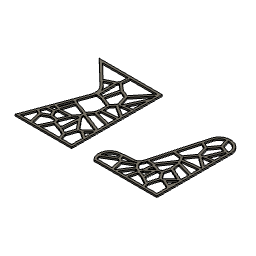
StrangeOutfit-Sides (Autodesk Fusion 360 design; units mm, degrees)
Autodesk Fusion 360 part; units mm, degrees
(part 1 of 2)
sketch "Sketch1" plane through (0, 0, 0) normal (0, 1, 0) x (1, 0, 0)
  line L0 (-508, 0) -> (0, 0)
  line L1 (-561.4783, 808.976) -> (-349.2633, 603.2383)
  arc A0 (-565.2203, 812.8) -> (-561.4783, 808.976) centre (-490.7581, 881.9227) ccw
  line L2 (-324.7055, 495.0118) -> (-508, 0)
  line L3 (0, 812.8) -> (-565.2203, 812.8)
  arc A1 (-349.2633, 603.2383) -> (-324.7055, 495.0118) centre (-419.9835, 530.2916) cw
  line L4 (0, 0) -> (0, 812.8)
  spline S0 degree 3 poles (197.1979, -94.8264) (181.7287, -81.3513) (181.7287, -81.3513) (184.3434, -52.8038) knots 0 0 0 0 1 1 1 1
  spline S1 degree 3 poles (184.3434, -52.8038) (186.9581, -24.2563) (186.9581, -24.2563) (221.5677, -24.2563) knots 0 0 0 0 1 1 1 1
  spline S2 degree 3 poles (221.5677, -24.2563) (256.1772, -24.2563) (256.1772, -24.2563) (249.4808, -61.402) knots 0 0 0 0 1 1 1 1
  spline S3 degree 3 poles (249.4808, -61.402) (242.7844, -98.5476) (242.7844, -98.5476) (227.7258, -103.4246) knots 0 0 0 0 1 1 1 1
  spline S4 degree 3 poles (227.7258, -103.4246) (212.6672, -108.3015) (212.6672, -108.3015) (197.1979, -94.8264) knots 0 0 0 0 1 1 1 1
  spline S5 degree 3 poles (314.1363, -605.8547) (333.9886, -586.6079) (333.9886, -586.6079) (347.2933, -588.796) knots 0 0 0 0 1 1 1 1
  spline S6 degree 3 poles (347.2933, -588.796) (360.598, -590.9842) (360.598, -590.9842) (371.6807, -608.3365) knots 0 0 0 0 1 1 1 1
  spline S7 degree 3 poles (371.6807, -608.3365) (382.7633, -625.6888) (382.7633, -625.6888) (369.5852, -652.1299) knots 0 0 0 0 1 1 1 1
  spline S8 degree 3 poles (369.5852, -652.1299) (356.4071, -678.5711) (356.4071, -678.5711) (332.329, -676.3297) knots 0 0 0 0 1 1 1 1
  spline S9 degree 3 poles (332.329, -676.3297) (308.2508, -674.0883) (308.2508, -674.0883) (301.2674, -649.5949) knots 0 0 0 0 1 1 1 1
  spline S10 degree 3 poles (301.2674, -649.5949) (294.284, -625.1014) (294.284, -625.1014) (314.1363, -605.8546) knots 0 0 0 0 1 1 1 1
  line L5 (314.1363, -605.8546) -> (314.1363, -605.8547)
  spline S11 degree 3 poles (325.2577, -150.3081) (324.2502, -141.4606) (324.2502, -141.4606) (337.2456, -127.0451) knots 0 0 0 0 1 1 1 1
  spline S12 degree 3 poles (337.2456, -127.0451) (350.2411, -112.6297) (350.2411, -112.6297) (372.3999, -109.9629) knots 0 0 0 0 1 1 1 1
  spline S13 degree 3 poles (372.3999, -109.9629) (394.5588, -107.2962) (394.5588, -107.2962) (414.281, -123.2421) knots 0 0 0 0 1 1 1 1
  spline S14 degree 3 poles (414.281, -123.2421) (434.0032, -139.1881) (434.0032, -139.1881) (430.6769, -158.3617) knots 0 0 0 0 1 1 1 1
  spline S15 degree 3 poles (430.6769, -158.3617) (427.3505, -177.5353) (427.3505, -177.5353) (401.8439, -188.2391) knots 0 0 0 0 1 1 1 1
  spline S16 degree 3 poles (401.8439, -188.2391) (376.3374, -198.943) (376.3374, -198.943) (351.3013, -179.0493) knots 0 0 0 0 1 1 1 1
  spline S17 degree 3 poles (351.3013, -179.0493) (326.2652, -159.1556) (326.2652, -159.1556) (325.2577, -150.3081) knots 0 0 0 0 1 1 1 1
  spline S18 degree 3 poles (356.0613, -480.7521) (387.4233, -481.317) (387.4233, -481.317) (397.359, -499.3064) knots 0 0 0 0 1 1 1 1
  spline S19 degree 3 poles (397.359, -499.3064) (407.2948, -517.2958) (407.2948, -517.2958) (386.1882, -543.2085) knots 0 0 0 0 1 1 1 1
  spline S20 degree 3 poles (386.1882, -543.2085) (365.0816, -569.1212) (365.0816, -569.1212) (351.2654, -566.8489) knots 0 0 0 0 1 1 1 1
  spline S21 degree 3 poles (351.2654, -566.8489) (337.4492, -564.5766) (337.4492, -564.5766) (323.3468, -539.9771) knots 0 0 0 0 1 1 1 1
  spline S22 degree 3 poles (323.3468, -539.9771) (309.2444, -515.3777) (309.2444, -515.3777) (316.9719, -497.7824) knots 0 0 0 0 1 1 1 1
  spline S23 degree 3 poles (316.9719, -497.7824) (324.6994, -480.1871) (324.6994, -480.1871) (356.0613, -480.752) knots 0 0 0 0 1 1 1 1
  line L6 (356.0613, -480.752) -> (356.0613, -480.7521)
  spline S24 degree 3 poles (387.6685, -660.8912) (400.7266, -634.6908) (400.7266, -634.6908) (423.4349, -636.471) knots 0 0 0 0 1 1 1 1
  spline S25 degree 3 poles (423.4349, -636.471) (446.1432, -638.2512) (446.1432, -638.2512) (456.0097, -663.7671) knots 0 0 0 0 1 1 1 1
  spline S26 degree 3 poles (456.0097, -663.7671) (465.8762, -689.283) (465.8762, -689.283) (457.4993, -699.4999) knots 0 0 0 0 1 1 1 1
  spline S27 degree 3 poles (457.4993, -699.4999) (449.1223, -709.7169) (449.1223, -709.7169) (419.0273, -708.316) knots 0 0 0 0 1 1 1 1
  spline S28 degree 3 poles (419.0273, -708.316) (388.9322, -706.9152) (388.9322, -706.9152) (381.7713, -697.0034) knots 0 0 0 0 1 1 1 1
  spline S29 degree 3 poles (381.7713, -697.0034) (374.6104, -687.0917) (374.6104, -687.0917) (387.6685, -660.8913) knots 0 0 0 0 1 1 1 1
  line L7 (387.6685, -660.8913) -> (387.6685, -660.8912)
  spline S30 degree 3 poles (404.7879, -382.8824) (386.9787, -364.4613) (386.9787, -364.4613) (396.7831, -338.1032) knots 0 0 0 0 1 1 1 1
  spline S31 degree 3 poles (396.7831, -338.1032) (406.5874, -311.7451) (406.5874, -311.7451) (427.3969, -309.3698) knots 0 0 0 0 1 1 1 1
  spline S32 degree 3 poles (427.3969, -309.3698) (448.2065, -306.9944) (448.2065, -306.9944) (464.4713, -324.5012) knots 0 0 0 0 1 1 1 1
  spline S33 degree 3 poles (464.4713, -324.5012) (480.7362, -342.0079) (480.7362, -342.0079) (466.7089, -368.8424) knots 0 0 0 0 1 1 1 1
  spline S34 degree 3 poles (466.7089, -368.8424) (452.6817, -395.6768) (452.6817, -395.6768) (437.6393, -398.4902) knots 0 0 0 0 1 1 1 1
  spline S35 degree 3 poles (437.6393, -398.4902) (422.597, -401.3035) (422.597, -401.3035) (404.7878, -382.8824) knots 0 0 0 0 1 1 1 1
  line L8 (404.7878, -382.8824) -> (404.7879, -382.8824)
  spline S36 degree 3 poles (185.1347, -753.5733) (182.1571, -789.0148) (182.1571, -789.0148) (149.5573, -789.0148) knots 0 0 0 0 1 1 1 1
  spline S37 degree 3 poles (149.5573, -789.0148) (116.9575, -789.0148) (116.9575, -789.0148) (114.8929, -752.1146) knots 0 0 0 0 1 1 1 1
  spline S38 degree 3 poles (114.8929, -752.1146) (112.8282, -715.2145) (112.8282, -715.2145) (113.8529, -714.1235) knots 0 0 0 0 1 1 1 1
  spline S39 degree 3 poles (113.8529, -714.1235) (114.8777, -713.0325) (114.8777, -713.0325) (147.0962, -711.0195) knots 0 0 0 0 1 1 1 1
  spline S40 degree 3 poles (147.0962, -711.0195) (179.3148, -709.0066) (179.3148, -709.0066) (183.7135, -713.5691) knots 0 0 0 0 1 1 1 1
  spline S41 degree 3 poles (183.7135, -713.5691) (188.1122, -718.1316) (188.1122, -718.1316) (185.1347, -753.5732) knots 0 0 0 0 1 1 1 1
  line L9 (185.1347, -753.5732) -> (185.1347, -753.5733)
  spline S42 degree 3 poles (398.2716, -56.4462) (390.271, -88.5918) (390.271, -88.5918) (370.6111, -90.9578) knots 0 0 0 0 1 1 1 1
  spline S43 degree 3 poles (370.6111, -90.9578) (350.9513, -93.3237) (350.9513, -93.3237) (340.7662, -58.8122) knots 0 0 0 0 1 1 1 1
  spline S44 degree 3 poles (340.7662, -58.8122) (330.581, -24.3006) (330.581, -24.3006) (368.4266, -24.3006) knots 0 0 0 0 1 1 1 1
  spline S45 degree 3 poles (368.4266, -24.3006) (406.2722, -24.3006) (406.2722, -24.3006) (398.2716, -56.4462) knots 0 0 0 0 1 1 1 1
  line L10 (398.2716, -56.4462) -> (398.2716, -56.4462)
  spline S46 degree 3 poles (321.4781, -406.2143) (332.5431, -384.0384) (332.5431, -384.0384) (352.3085, -380.8845) knots 0 0 0 0 1 1 1 1
  spline S47 degree 3 poles (352.3085, -380.8845) (372.0739, -377.7306) (372.0739, -377.7306) (389.7648, -396.0293) knots 0 0 0 0 1 1 1 1
  spline S48 degree 3 poles (389.7648, -396.0293) (407.4556, -414.3281) (407.4556, -414.3281) (397.2221, -437.6806) knots 0 0 0 0 1 1 1 1
  spline S49 degree 3 poles (397.2221, -437.6806) (386.9886, -461.0332) (386.9886, -461.0332) (356.2186, -460.479) knots 0 0 0 0 1 1 1 1
  spline S50 degree 3 poles (356.2186, -460.479) (325.4486, -459.9247) (325.4486, -459.9247) (317.9308, -444.1575) knots 0 0 0 0 1 1 1 1
  spline S51 degree 3 poles (317.9308, -444.1575) (310.4131, -428.3902) (310.4131, -428.3902) (321.4781, -406.2144) knots 0 0 0 0 1 1 1 1
  line L11 (321.4781, -406.2144) -> (321.4781, -406.2143)
  spline S52 degree 3 poles (264.9537, -529.8005) (293.6396, -524.3322) (293.6396, -524.3322) (307.4969, -548.5041) knots 0 0 0 0 1 1 1 1
  spline S53 degree 3 poles (307.4969, -548.5041) (321.3541, -572.676) (321.3541, -572.676) (301.097, -592.3153) knots 0 0 0 0 1 1 1 1
  spline S54 degree 3 poles (301.097, -592.3153) (280.8398, -611.9546) (280.8398, -611.9546) (257.4922, -604.1541) knots 0 0 0 0 1 1 1 1
  spline S55 degree 3 poles (257.4922, -604.1541) (234.1447, -596.3536) (234.1447, -596.3536) (235.2062, -565.8113) knots 0 0 0 0 1 1 1 1
  spline S56 degree 3 poles (235.2062, -565.8113) (236.2677, -535.2689) (236.2677, -535.2689) (264.9537, -529.8005) knots 0 0 0 0 1 1 1 1
  spline S57 degree 3 poles (380.3364, -237.5005) (384.7414, -214.6927) (384.7414, -214.6927) (409.0824, -204.478) knots 0 0 0 0 1 1 1 1
  spline S58 degree 3 poles (409.0824, -204.478) (433.4234, -194.2633) (433.4234, -194.2633) (450.4003, -212.6655) knots 0 0 0 0 1 1 1 1
  spline S59 degree 3 poles (450.4003, -212.6655) (467.377, -231.0678) (467.377, -231.0678) (456.5522, -258.126) knots 0 0 0 0 1 1 1 1
  spline S60 degree 3 poles (456.5522, -258.126) (445.7273, -285.1843) (445.7273, -285.1843) (424.898, -287.5619) knots 0 0 0 0 1 1 1 1
  spline S61 degree 3 poles (424.898, -287.5619) (404.0687, -289.9394) (404.0687, -289.9394) (390, -275.1238) knots 0 0 0 0 1 1 1 1
  spline S62 degree 3 poles (390, -275.1238) (375.9314, -260.3082) (375.9314, -260.3082) (380.3364, -237.5005) knots 0 0 0 0 1 1 1 1
  spline S63 degree 3 poles (518.1162, -109.8607) (490.6468, -105.3557) (490.6468, -105.3557) (487.0263, -64.3304) knots 0 0 0 0 1 1 1 1
  spline S64 degree 3 poles (487.0263, -64.3304) (483.4058, -23.305) (483.4058, -23.305) (514.4957, -23.305) knots 0 0 0 0 1 1 1 1
  spline S65 degree 3 poles (514.4957, -23.305) (545.5855, -23.305) (545.5855, -23.305) (545.5855, -68.8354) knots 0 0 0 0 1 1 1 1
  spline S66 degree 3 poles (545.5855, -68.8354) (545.5855, -114.3657) (545.5855, -114.3657) (518.1162, -109.8607) knots 0 0 0 0 1 1 1 1
  spline S67 degree 3 poles (441.522, -418.9688) (457.0203, -416.0701) (457.0203, -416.0701) (483.5167, -439.8327) knots 0 0 0 0 1 1 1 1
  spline S68 degree 3 poles (483.5167, -439.8327) (510.0132, -463.5952) (510.0132, -463.5952) (483.0172, -488.7104) knots 0 0 0 0 1 1 1 1
  spline S69 degree 3 poles (483.0172, -488.7104) (456.0211, -513.8256) (456.0211, -513.8256) (440.5191, -510.3742) knots 0 0 0 0 1 1 1 1
  spline S70 degree 3 poles (440.5191, -510.3742) (425.0171, -506.9227) (425.0171, -506.9227) (414.9062, -488.6162) knots 0 0 0 0 1 1 1 1
  spline S71 degree 3 poles (414.9062, -488.6162) (404.7954, -470.3098) (404.7954, -470.3098) (415.4095, -446.0886) knots 0 0 0 0 1 1 1 1
  spline S72 degree 3 poles (415.4095, -446.0886) (426.0237, -421.8674) (426.0237, -421.8674) (441.522, -418.9688) knots 0 0 0 0 1 1 1 1
  spline S73 degree 3 poles (474.2518, -266.1599) (484.6175, -240.2495) (484.6175, -240.2495) (513.0731, -237.6245) knots 0 0 0 0 1 1 1 1
  spline S74 degree 3 poles (513.0731, -237.6245) (541.5287, -234.9996) (541.5287, -234.9996) (541.5287, -279.1463) knots 0 0 0 0 1 1 1 1
  spline S75 degree 3 poles (541.5287, -279.1463) (541.5287, -323.293) (541.5287, -323.293) (518.2971, -324.4617) knots 0 0 0 0 1 1 1 1
  spline S76 degree 3 poles (518.2971, -324.4617) (495.0655, -325.6304) (495.0655, -325.6304) (479.4758, -308.8504) knots 0 0 0 0 1 1 1 1
  spline S77 degree 3 poles (479.4758, -308.8504) (463.8861, -292.0704) (463.8861, -292.0704) (474.2518, -266.1599) knots 0 0 0 0 1 1 1 1
  spline S78 degree 3 poles (532.861, -454.3391) (519.4812, -454.2704) (519.4812, -454.2704) (492.0593, -429.6779) knots 0 0 0 0 1 1 1 1
  spline S79 degree 3 poles (492.0593, -429.6779) (464.6374, -405.0854) (464.6374, -405.0854) (479.5946, -376.472) knots 0 0 0 0 1 1 1 1
  spline S80 degree 3 poles (479.5946, -376.472) (494.5517, -347.8586) (494.5517, -347.8586) (520.3962, -346.5584) knots 0 0 0 0 1 1 1 1
  spline S81 degree 3 poles (520.3962, -346.5584) (546.2408, -345.2582) (546.2408, -345.2582) (546.2408, -399.833) knots 0 0 0 0 1 1 1 1
  spline S82 degree 3 poles (546.2408, -399.833) (546.2408, -454.4078) (546.2408, -454.4078) (532.861, -454.3391) knots 0 0 0 0 1 1 1 1
  line L12 (532.861, -454.3391) -> (532.861, -454.3391)
  spline S83 degree 3 poles (287.1401, -246.3243) (272.1959, -224.4344) (272.1959, -224.4344) (294.6473, -198.5119) knots 0 0 0 0 1 1 1 1
  spline S84 degree 3 poles (294.6473, -198.5119) (317.0987, -172.5894) (317.0987, -172.5894) (340.9663, -191.5547) knots 0 0 0 0 1 1 1 1
  spline S85 degree 3 poles (340.9663, -191.5547) (364.834, -210.5199) (364.834, -210.5199) (360.4335, -233.3043) knots 0 0 0 0 1 1 1 1
  spline S86 degree 3 poles (360.4335, -233.3043) (356.033, -256.0887) (356.033, -256.0887) (329.0586, -262.1515) knots 0 0 0 0 1 1 1 1
  spline S87 degree 3 poles (329.0586, -262.1515) (302.0843, -268.2142) (302.0843, -268.2142) (287.1401, -246.3243) knots 0 0 0 0 1 1 1 1
  spline S88 degree 3 poles (165.1478, -50.93) (162.5663, -79.1146) (162.5663, -79.1146) (135.0164, -86.2518) knots 0 0 0 0 1 1 1 1
  spline S89 degree 3 poles (135.0164, -86.2518) (107.4664, -93.389) (107.4664, -93.389) (100.4948, -58.0672) knots 0 0 0 0 1 1 1 1
  spline S90 degree 3 poles (100.4948, -58.0672) (93.5233, -22.7453) (93.5233, -22.7453) (130.6263, -22.7453) knots 0 0 0 0 1 1 1 1
  spline S91 degree 3 poles (130.6263, -22.7453) (167.7293, -22.7453) (167.7293, -22.7453) (165.1478, -50.93) knots 0 0 0 0 1 1 1 1
  spline S92 degree 3 poles (510.251, -790.3275) (476.5909, -790.3275) (476.5909, -790.3275) (471.5964, -757.9443) knots 0 0 0 0 1 1 1 1
  spline S93 degree 3 poles (471.5964, -757.9443) (466.6018, -725.5611) (466.6018, -725.5611) (475.3691, -714.868) knots 0 0 0 0 1 1 1 1
  spline S94 degree 3 poles (475.3691, -714.868) (484.1365, -704.1748) (484.1365, -704.1748) (514.0238, -704.5036) knots 0 0 0 0 1 1 1 1
  spline S95 degree 3 poles (514.0238, -704.5036) (543.911, -704.8323) (543.911, -704.8323) (543.911, -747.5799) knots 0 0 0 0 1 1 1 1
  spline S96 degree 3 poles (543.911, -747.5799) (543.911, -790.3275) (543.911, -790.3275) (510.251, -790.3275) knots 0 0 0 0 1 1 1 1
  spline S97 degree 3 poles (280.9941, -655.0186) (288.0544, -679.7817) (288.0544, -679.7817) (279.2804, -689.2798) knots 0 0 0 0 1 1 1 1
  spline S98 degree 3 poles (279.2804, -689.2798) (270.5063, -698.778) (270.5063, -698.778) (239.3092, -698.6341) knots 0 0 0 0 1 1 1 1
  spline S99 degree 3 poles (239.3092, -698.6341) (208.1122, -698.4901) (208.1122, -698.4901) (203.6413, -693.8528) knots 0 0 0 0 1 1 1 1
  spline S100 degree 3 poles (203.6413, -693.8528) (199.1703, -689.2154) (199.1703, -689.2154) (202.7198, -658.8368) knots 0 0 0 0 1 1 1 1
  spline S101 degree 3 poles (202.7198, -658.8368) (206.2693, -628.4583) (206.2693, -628.4583) (216.9688, -621.6282) knots 0 0 0 0 1 1 1 1
  spline S102 degree 3 poles (216.9688, -621.6282) (227.6682, -614.7981) (227.6682, -614.7981) (250.801, -622.5268) knots 0 0 0 0 1 1 1 1
  spline S103 degree 3 poles (250.801, -622.5268) (273.9338, -630.2556) (273.9338, -630.2556) (280.9941, -655.0187) knots 0 0 0 0 1 1 1 1
  line L13 (280.9941, -655.0187) -> (280.9941, -655.0186)
  spline S104 degree 3 poles (299.7019, -303.8393) (305.7178, -287.0219) (305.7178, -287.0219) (333.1511, -280.8561) knots 0 0 0 0 1 1 1 1
  spline S105 degree 3 poles (333.1511, -280.8561) (360.5844, -274.6902) (360.5844, -274.6902) (374.8778, -289.7425) knots 0 0 0 0 1 1 1 1
  spline S106 degree 3 poles (374.8778, -289.7425) (389.1712, -304.7948) (389.1712, -304.7948) (379.2008, -331.5994) knots 0 0 0 0 1 1 1 1
  spline S107 degree 3 poles (379.2008, -331.5994) (369.2304, -358.4041) (369.2304, -358.4041) (348.9957, -361.6329) knots 0 0 0 0 1 1 1 1
  spline S108 degree 3 poles (348.9957, -361.6329) (328.761, -364.8617) (328.761, -364.8617) (311.2235, -342.7592) knots 0 0 0 0 1 1 1 1
  spline S109 degree 3 poles (311.2235, -342.7592) (293.686, -320.6566) (293.686, -320.6566) (299.7019, -303.8393) knots 0 0 0 0 1 1 1 1
  line L14 (299.7019, -303.8393) -> (299.7019, -303.8393)
  spline S110 degree 3 poles (518.412, -576.7998) (491.3849, -575.5092) (491.3849, -575.5092) (477.8348, -549.8725) knots 0 0 0 0 1 1 1 1
  spline S111 degree 3 poles (477.8348, -549.8725) (464.2848, -524.2357) (464.2848, -524.2357) (491.7223, -498.7098) knots 0 0 0 0 1 1 1 1
  spline S112 degree 3 poles (491.7223, -498.7098) (519.1598, -473.1839) (519.1598, -473.1839) (532.2995, -473.2513) knots 0 0 0 0 1 1 1 1
  spline S113 degree 3 poles (532.2995, -473.2513) (545.4391, -473.3188) (545.4391, -473.3188) (545.4391, -525.7046) knots 0 0 0 0 1 1 1 1
  spline S114 degree 3 poles (545.4391, -525.7046) (545.4391, -578.0904) (545.4391, -578.0904) (518.412, -576.7998) knots 0 0 0 0 1 1 1 1
  spline S115 degree 3 poles (215.9507, -192.8402) (204.8811, -174.279) (204.8811, -174.279) (211.9244, -151.2755) knots 0 0 0 0 1 1 1 1
  spline S116 degree 3 poles (211.9244, -151.2755) (218.9678, -128.272) (218.9678, -128.272) (234.8773, -123.1195) knots 0 0 0 0 1 1 1 1
  spline S117 degree 3 poles (234.8773, -123.1195) (250.7869, -117.967) (250.7869, -117.967) (277.4311, -131.0928) knots 0 0 0 0 1 1 1 1
  spline S118 degree 3 poles (277.4311, -131.0928) (304.0753, -144.2186) (304.0753, -144.2186) (305.065, -152.9095) knots 0 0 0 0 1 1 1 1
  spline S119 degree 3 poles (305.065, -152.9095) (306.0546, -161.6005) (306.0546, -161.6005) (282.9209, -188.3107) knots 0 0 0 0 1 1 1 1
  spline S120 degree 3 poles (282.9209, -188.3107) (259.7872, -215.021) (259.7872, -215.021) (243.4038, -213.2112) knots 0 0 0 0 1 1 1 1
  spline S121 degree 3 poles (243.4038, -213.2112) (227.0204, -211.4014) (227.0204, -211.4014) (215.9507, -192.8402) knots 0 0 0 0 1 1 1 1
  spline S122 degree 3 poles (205.0633, -754.7842) (208.052, -719.2098) (208.052, -719.2098) (238.8605, -719.3519) knots 0 0 0 0 1 1 1 1
  spline S123 degree 3 poles (238.8605, -719.3519) (269.6689, -719.494) (269.6689, -719.494) (275.1957, -754.9263) knots 0 0 0 0 1 1 1 1
  spline S124 degree 3 poles (275.1957, -754.9263) (280.7225, -790.3586) (280.7225, -790.3586) (241.3985, -790.3586) knots 0 0 0 0 1 1 1 1
  spline S125 degree 3 poles (241.3985, -790.3586) (202.0746, -790.3586) (202.0746, -790.3586) (205.0633, -754.7842) knots 0 0 0 0 1 1 1 1
  spline S126 degree 3 poles (363.3588, -710.9786) (370.9858, -721.5356) (370.9858, -721.5356) (363.7449, -755.9828) knots 0 0 0 0 1 1 1 1
  spline S127 degree 3 poles (363.7449, -755.9828) (356.5041, -790.43) (356.5041, -790.43) (327.3888, -790.43) knots 0 0 0 0 1 1 1 1
  spline S128 degree 3 poles (327.3888, -790.43) (298.2736, -790.43) (298.2736, -790.43) (292.4313, -752.9754) knots 0 0 0 0 1 1 1 1
  spline S129 degree 3 poles (292.4313, -752.9754) (286.5891, -715.5208) (286.5891, -715.5208) (295.7484, -705.6057) knots 0 0 0 0 1 1 1 1
  spline S130 degree 3 poles (295.7484, -705.6057) (304.9077, -695.6905) (304.9077, -695.6905) (330.3197, -698.0561) knots 0 0 0 0 1 1 1 1
  spline S131 degree 3 poles (330.3197, -698.0561) (355.7317, -700.4216) (355.7317, -700.4216) (363.3588, -710.9786) knots 0 0 0 0 1 1 1 1
  line L15 (363.3588, -710.9786) -> (363.3588, -710.9786)
  spline S132 degree 3 poles (417.1745, -60.4217) (425.0552, -28.7577) (425.0552, -28.7577) (445.9853, -28.7577) knots 0 0 0 0 1 1 1 1
  spline S133 degree 3 poles (445.9853, -28.7577) (466.9153, -28.7577) (466.9153, -28.7577) (470.2084, -66.0731) knots 0 0 0 0 1 1 1 1
  spline S134 degree 3 poles (470.2084, -66.0731) (473.5015, -103.3884) (473.5015, -103.3884) (458.6335, -111.6726) knots 0 0 0 0 1 1 1 1
  spline S135 degree 3 poles (458.6335, -111.6726) (443.7654, -119.9569) (443.7654, -119.9569) (426.5296, -106.0213) knots 0 0 0 0 1 1 1 1
  spline S136 degree 3 poles (426.5296, -106.0213) (409.2938, -92.0856) (409.2938, -92.0856) (417.1745, -60.4217) knots 0 0 0 0 1 1 1 1
  line L16 (417.1745, -60.4217) -> (417.1745, -60.4217)
  spline S137 degree 3 poles (381.1017, -758.7245) (387.9376, -726.2041) (387.9376, -726.2041) (418.1988, -727.6126) knots 0 0 0 0 1 1 1 1
  spline S138 degree 3 poles (418.1988, -727.6126) (448.46, -729.0212) (448.46, -729.0212) (453.2585, -760.133) knots 0 0 0 0 1 1 1 1
  spline S139 degree 3 poles (453.2585, -760.133) (458.0571, -791.2449) (458.0571, -791.2449) (416.1614, -791.2449) knots 0 0 0 0 1 1 1 1
  spline S140 degree 3 poles (416.1614, -791.2449) (374.2658, -791.2449) (374.2658, -791.2449) (381.1017, -758.7245) knots 0 0 0 0 1 1 1 1
  spline S141 degree 3 poles (517.7573, -596.1784) (544.1556, -597.439) (544.1556, -597.439) (544.1556, -641.3222) knots 0 0 0 0 1 1 1 1
  spline S142 degree 3 poles (544.1556, -641.3222) (544.1556, -685.2055) (544.1556, -685.2055) (513.9239, -684.8729) knots 0 0 0 0 1 1 1 1
  spline S143 degree 3 poles (513.9239, -684.8729) (483.6922, -684.5404) (483.6922, -684.5404) (473.2467, -657.5273) knots 0 0 0 0 1 1 1 1
  spline S144 degree 3 poles (473.2467, -657.5273) (462.8013, -630.5142) (462.8013, -630.5142) (477.0802, -612.7161) knots 0 0 0 0 1 1 1 1
  spline S145 degree 3 poles (477.0802, -612.7161) (491.359, -594.9179) (491.359, -594.9179) (517.7573, -596.1784) knots 0 0 0 0 1 1 1 1
  line L17 (517.7573, -596.1784) -> (517.7573, -596.1784)
  spline S146 degree 3 poles (261.1625, -435.5885) (289.8221, -439.4724) (289.8221, -439.4724) (297.2993, -455.1546) knots 0 0 0 0 1 1 1 1
  spline S147 degree 3 poles (297.2993, -455.1546) (304.7765, -470.8368) (304.7765, -470.8368) (297.2358, -488.0067) knots 0 0 0 0 1 1 1 1
  spline S148 degree 3 poles (297.2358, -488.0067) (289.6951, -505.1767) (289.6951, -505.1767) (261.2073, -510.6073) knots 0 0 0 0 1 1 1 1
  spline S149 degree 3 poles (261.2073, -510.6073) (232.7195, -516.0379) (232.7195, -516.0379) (223.151, -507.8695) knots 0 0 0 0 1 1 1 1
  spline S150 degree 3 poles (223.151, -507.8695) (213.5824, -499.7011) (213.5824, -499.7011) (212.5904, -476.2029) knots 0 0 0 0 1 1 1 1
  spline S151 degree 3 poles (212.5904, -476.2029) (211.5984, -452.7048) (211.5984, -452.7048) (222.0507, -442.2047) knots 0 0 0 0 1 1 1 1
  spline S152 degree 3 poles (222.0507, -442.2047) (232.503, -431.7045) (232.503, -431.7045) (261.1625, -435.5885) knots 0 0 0 0 1 1 1 1
  spline S153 degree 3 poles (284.8449, -114.0737) (258.8484, -101.267) (258.8484, -101.267) (265.7512, -62.9764) knots 0 0 0 0 1 1 1 1
  spline S154 degree 3 poles (265.7512, -62.9764) (272.654, -24.6858) (272.654, -24.6858) (293.2004, -24.6858) knots 0 0 0 0 1 1 1 1
  spline S155 degree 3 poles (293.2004, -24.6858) (313.7467, -24.6858) (313.7467, -24.6858) (324.7493, -61.9669) knots 0 0 0 0 1 1 1 1
  spline S156 degree 3 poles (324.7493, -61.9669) (335.7518, -99.2481) (335.7518, -99.2481) (323.2966, -113.0643) knots 0 0 0 0 1 1 1 1
  spline S157 degree 3 poles (323.2966, -113.0643) (310.8415, -126.8804) (310.8415, -126.8804) (284.8449, -114.0737) knots 0 0 0 0 1 1 1 1
  spline S158 degree 3 poles (450.2166, -161.6307) (453.4652, -142.9053) (453.4652, -142.9053) (470.0804, -133.6475) knots 0 0 0 0 1 1 1 1
  spline S159 degree 3 poles (470.0804, -133.6475) (486.6956, -124.3898) (486.6956, -124.3898) (514.6169, -128.9689) knots 0 0 0 0 1 1 1 1
  spline S160 degree 3 poles (514.6169, -128.9689) (542.5382, -133.5481) (542.5382, -133.5481) (542.5382, -172.9795) knots 0 0 0 0 1 1 1 1
  spline S161 degree 3 poles (542.5382, -172.9795) (542.5382, -212.4109) (542.5382, -212.4109) (512.127, -215.2162) knots 0 0 0 0 1 1 1 1
  spline S162 degree 3 poles (512.127, -215.2162) (481.7157, -218.0215) (481.7157, -218.0215) (464.3419, -199.1888) knots 0 0 0 0 1 1 1 1
  spline S163 degree 3 poles (464.3419, -199.1888) (446.968, -180.3562) (446.968, -180.3562) (450.2166, -161.6307) knots 0 0 0 0 1 1 1 1
  spline S164 degree 3 poles (435.6277, -529.7216) (450.8638, -533.1139) (450.8638, -533.1139) (463.9671, -557.9055) knots 0 0 0 0 1 1 1 1
  spline S165 degree 3 poles (463.9671, -557.9055) (477.0704, -582.6971) (477.0704, -582.6971) (462.9334, -600.3185) knots 0 0 0 0 1 1 1 1
  spline S166 degree 3 poles (462.9334, -600.3185) (448.7964, -617.9399) (448.7964, -617.9399) (424.9945, -616.074) knots 0 0 0 0 1 1 1 1
  spline S167 degree 3 poles (424.9945, -616.074) (401.1926, -614.208) (401.1926, -614.208) (389.682, -596.1857) knots 0 0 0 0 1 1 1 1
  spline S168 degree 3 poles (389.682, -596.1857) (378.1714, -578.1633) (378.1714, -578.1633) (399.2815, -552.2463) knots 0 0 0 0 1 1 1 1
  spline S169 degree 3 poles (399.2815, -552.2463) (420.3916, -526.3293) (420.3916, -526.3293) (435.6277, -529.7216) knots 0 0 0 0 1 1 1 1
sketch "Sketch2" plane through (0, 0, 0) normal (0, 1, 0) x (1, 0, 0)
  arc A0 (426.5564, 220.9132) -> (380.9487, 182.765) centre (376.1491, 234.8401) cw
  line L0 (762.7191, 1.5665) -> (762.7191, 667.0349)
  arc A1 (762.7191, 667.0349) -> (662.5091, 768.6254) centre (661.1191, 667.0349) ccw
  arc A2 (656.633, 768.7058) -> (557.312, 694.1724) centre (655.2429, 667.1153) ccw
  arc A3 (262.6363, 171.8604) -> (197.4988, 1.5665) centre (271.961, 70.6892) ccw
  line L1 (380.9487, 182.765) -> (262.6363, 171.8604)
  line L2 (557.312, 694.1724) -> (426.5564, 220.9132)
  line L3 (662.5091, 768.6254) -> (656.633, 768.7058)
  line L4 (197.4988, 1.5665) -> (762.7191, 1.5665)
sketch "Voronoi Sketch" plane through (0, 0, 0) normal (0, 1, 0) x (1, 0, 0)
  line L0 (644.2098, 519.254) -> (660.307, 524.9005)
  line L1 (664.2606, 528.6756) -> (712.3302, 647.7946)
  line L2 (710.6678, 651.6916) -> (675.4495, 665.7911)
  line L3 (670.8923, 664.4854) -> (621.1441, 596.5326)
  line L4 (620.2079, 591.2308) -> (640.543, 521.1422)
  line L5 (542.0247, 106.9356) -> (546.4509, 166.1735)
  line L6 (544.4555, 167.1462) -> (510.039, 135.8306)
  line L7 (505.999, 131.4276) -> (497.0019, 119.6492)
  line L8 (497.3996, 119.0298) -> (538.9606, 104.9091)
  line L9 (516.3543, 168.617) -> (550.0484, 199.2752)
  line L10 (551.1464, 202.4274) -> (523.4858, 212.5174)
  line L11 (520.2541, 210.574) -> (514.5488, 169.5694)
  line L12 (518.383, 235.6679) -> (565.6759, 218.4164)
  line L13 (571.4272, 218.0193) -> (587.4541, 221.4671)
  line L14 (591.1381, 225.0026) -> (605.3824, 280.0857)
  line L15 (605.7019, 285.9589) -> (595.8422, 353.775)
  line L16 (594.1769, 355.4648) -> (514.844, 239.3873)
  line L17 (622.2982, 265.6147) -> (610.1441, 218.6145)
  line L18 (611.1678, 213.2913) -> (646.3219, 165.3826)
  line L19 (650.9437, 163.9096) -> (659.4472, 166.7341)
  line L20 (664.3899, 169.8264) -> (717.0837, 223.8031)
  line L21 (716.4363, 227.1645) -> (625.7924, 267.3045)
  line L22 (591.3606, 201.85) -> (576.7137, 198.699)
  line L23 (572.0877, 195.5915) -> (569.9828, 192.5127)
  line L24 (568.0661, 187.0445) -> (561.488, 99.0072)
  line L25 (563.8992, 94.5808) -> (607.161, 71.0227)
  line L26 (610.6461, 72.4649) -> (632.4953, 146.3829)
  line L27 (631.5709, 151.6786) -> (596.0683, 200.0622)
  line L28 (343.6418, 100.6753) -> (359.1998, 24.5058)
  line L29 (362.8002, 21.5665) -> (369.3723, 21.5665)
  line L30 (373.9863, 24.0953) -> (440.2889, 127.9828)
  line L31 (439.9093, 132.7535) -> (424.6176, 149.9496)
  line L32 (420.0634, 150.6284) -> (345.6021, 105.1777)
  line L33 (399.0984, 21.5665) -> (456.1374, 21.5665)
  line L34 (459.859, 24.4784) -> (480.0308, 105.8825)
  line L35 (476.1489, 111.3823) -> (461.0356, 117.8144)
  line L36 (456.6612, 116.4603) -> (397.7124, 24.0953)
  line L37 (482.7423, 21.5665) -> (612.5479, 21.5665)
  line L38 (614.6761, 24.437) -> (608.3719, 45.1945)
  line L39 (604.8654, 49.4997) -> (549.4168, 79.6941)
  line L40 (543.9415, 82.0939) -> (501.402, 96.5471)
  line L41 (497.8399, 94.6002) -> (480.4639, 24.4784)
  line L42 (742.7191, 24.5665) -> (742.7191, 106.5435)
  line L43 (740.3296, 111.3574) -> (729.4931, 119.5832)
  line L44 (724.3659, 122.624) -> (669.9503, 147.0121)
  line L45 (664.3656, 147.2934) -> (655.297, 144.2811)
  line L46 (651.5996, 140.4585) -> (627.1682, 57.8049)
  line L47 (627.1896, 52.0574) -> (635.5782, 24.437)
  line L48 (639.45, 21.5665) -> (739.7191, 21.5665)
  line L49 (741.5615, 220.2462) -> (687.0116, 164.3682)
  line L50 (687.6536, 160.9946) -> (723.2394, 145.0457)
  line L51 (726.8512, 146.6886) -> (741.845, 195.9124)
  line L52 (742.7191, 201.7822) -> (742.7191, 220.4063)
  line L53 (628.1633, 288.1278) -> (734.1279, 241.2034)
  line L54 (739.7116, 240.9533) -> (739.8784, 241.0099)
  line L55 (742.7191, 244.9746) -> (742.7191, 305.7112)
  line L56 (739.8343, 309.5344) -> (620.2902, 343.6464)
  line L57 (617.837, 341.5008) -> (624.9886, 292.3113)
  line L58 (604.7133, 377.3815) -> (609.9478, 369.4309)
  line L59 (614.4823, 366.102) -> (739.8343, 330.3328)
  line L60 (742.7191, 332.5096) -> (742.7191, 394.3219)
  line L61 (739.7358, 397.0058) -> (604.0386, 382.628)
  line L62 (583.4238, 413.8766) -> (590.5272, 403.9342)
  line L63 (595.2545, 401.8092) -> (740.1772, 417.1645)
  line L64 (740.653, 424.0511) -> (642.4132, 495.6115)
  line L65 (638.2365, 494.9425) -> (583.4317, 418.753)
  line L66 (742.7191, 450.2896) -> (742.7191, 514.9727)
  line L67 (739.7483, 517.5553) -> (676.0626, 508.6078)
  line L68 (670.2609, 507.1974) -> (666.4875, 505.8738)
  line L69 (666.0815, 503.1144) -> (740.2942, 449.056)
  line L70 (739.7401, 644.486) -> (735.8698, 644.9462)
  line L71 (731.7682, 642.5184) -> (687.5923, 533.0484)
  line L72 (689.4404, 530.6837) -> (739.7483, 537.7517)
  line L73 (742.7191, 541.1691) -> (742.7191, 641.1318)
  arc A0 (742.7191, 667.0349) -> (662.2355, 748.6273) centre (661.1191, 667.0349) ccw
  line L74 (662.2355, 748.6273) -> (656.3594, 748.7077)
  arc A1 (656.3594, 748.7077) -> (656.1628, 748.7102) centre (655.2429, 667.1153) ccw
  line L75 (656.0297, 748.5263) -> (676.1888, 689.4893)
  line L76 (679.9433, 685.5352) -> (726.1851, 667.0226)
  line L77 (731.9492, 665.5533) -> (741.3477, 664.4358)
  line L78 (742.7191, 665.6538) -> (742.7191, 667.0349)
  line L79 (563.0411, 628.7146) -> (602.5106, 609.9271)
  line L80 (606.9916, 611.0584) -> (656.2586, 678.3539)
  line L81 (657.0613, 683.6136) -> (636.6347, 743.4339)
  arc A2 (632.6322, 745.5202) -> (576.5897, 688.8462) centre (655.2429, 667.1153) ccw
  line L82 (576.5897, 688.8462) -> (561.1313, 632.8956)
  line L83 (566.4344, 429.3734) -> (621.6245, 506.0985)
  line L84 (622.5404, 511.415) -> (600.8806, 586.0695)
  line L85 (597.3359, 590.2401) -> (557.6326, 609.1389)
  line L86 (554.1249, 607.5366) -> (506.8748, 436.5188)
  line L87 (509.0566, 433.287) -> (561.7019, 427.2783)
  line L88 (496.3653, 247.7948) -> (581.7776, 372.7675)
  line L89 (582.2687, 377.9931) -> (579.9825, 383.2224)
  line L90 (577.0369, 388.4122) -> (565.5679, 404.4652)
  line L91 (560.8432, 407.2464) -> (503.6649, 413.7725)
  line L92 (499.8854, 411.221) -> (455.7575, 251.5037)
  line L93 (457.9483, 248.3641) -> (491.6828, 245.566)
  line L94 (432.4739, 186.2557) -> (433.8731, 172.2873)
  line L95 (436.1657, 167.0604) -> (458.3883, 142.0703)
  line L96 (463.1422, 138.6537) -> (477.897, 132.3743)
  line L97 (482.4785, 133.5835) -> (489.0583, 142.1974)
  line L98 (491.2928, 147.5528) -> (501.2387, 219.0357)
  line L99 (499.0794, 223.5501) -> (499.0712, 223.5549)
  line L100 (493.5087, 225.3459) -> (452.5278, 228.745)
  line L101 (448.7391, 226.1013) -> (445.8341, 215.587)
  arc A3 (433.8983, 191.3463) -> (445.8341, 215.587) centre (376.1491, 234.8401) ccw
  line L102 (305.0939, 152.7557) -> (310.1898, 137.4931)
  line L103 (313.6212, 132.9614) -> (329.6477, 122.0713)
  line L104 (334.6897, 121.9482) -> (412.8018, 169.6274)
  arc A4 (382.7843, 162.8494) -> (412.5284, 172.3642) centre (376.1491, 234.8401) ccw
  line L105 (382.7843, 162.8494) -> (307.1311, 155.8766)
  line L106 (193.0344, 74.6849) -> (288.1088, 131.2188)
  line L107 (289.7373, 135.5977) -> (284.6381, 150.8703)
  line L108 (280.7006, 153.4406) -> (264.4718, 151.9448)
  arc A5 (264.4718, 151.9448) -> (190.5482, 76.2128) centre (271.961, 70.6892) ccw
  line L109 (209.8758, 21.5665) -> (336.3872, 21.5665)
  line L110 (338.7869, 24.5058) -> (323.4552, 99.5674)
  line L111 (320.3734, 104.1928) -> (304.8483, 114.7423)
  line L112 (299.7884, 114.8951) -> (195.3461, 52.7908)
  arc A6 (193.5231, 48.1935) -> (204.9317, 24.1527) centre (271.961, 70.6892) ccw
  arc A7 (640.543, 521.1422) -> (644.2098, 519.254) centre (643.27, 521.9333) ccw
  arc A8 (660.307, 524.9005) -> (664.2606, 528.6756) centre (658.1125, 531.1566) ccw
  arc A9 (712.3302, 647.7946) -> (710.6678, 651.6916) centre (709.5559, 648.9142) ccw
  arc A10 (675.4495, 665.7911) -> (670.8923, 664.4854) centre (674.0124, 662.2012) ccw
  arc A11 (621.1441, 596.5326) -> (620.2079, 591.2308) centre (626.0649, 592.9301) ccw
  arc A12 (497.0019, 119.6492) -> (497.0161, 119.2833) centre (497.2301, 119.4748) ccw
  arc A13 (497.0161, 119.2833) -> (497.3996, 119.0298) centre (497.6909, 119.8872) ccw
  arc A14 (510.039, 135.8306) -> (505.999, 131.4276) centre (532.3839, 111.273) ccw
  arc A15 (538.9606, 104.9091) -> (542.0247, 106.9356) centre (539.708, 107.1087) ccw
  arc A16 (546.4509, 166.1735) -> (544.4555, 167.1462) centre (545.2596, 166.2625) ccw
  arc A17 (551.5898, 201.0465) -> (551.1464, 202.4274) centre (550.8318, 201.5647) ccw
  arc A18 (550.0484, 199.2752) -> (551.5898, 201.0465) centre (543.2466, 206.7505) ccw
  arc A19 (523.4858, 212.5174) -> (520.2541, 210.574) centre (522.6551, 210.24) ccw
  arc A20 (514.5488, 169.5694) -> (516.3543, 168.617) centre (515.6238, 169.4198) ccw
  arc A21 (595.8422, 353.775) -> (595.2032, 355.4559) centre (591.7454, 353.1794) ccw
  arc A22 (595.2032, 355.4559) -> (594.1769, 355.4648) centre (594.687, 355.1161) ccw
  arc A23 (514.844, 239.3873) -> (515.3406, 237.1188) centre (516.1612, 238.487) ccw
  arc A24 (515.3406, 237.1188) -> (518.383, 235.6679) centre (524.4577, 252.3208) ccw
  arc A25 (565.6759, 218.4164) -> (571.4272, 218.0193) centre (569.2399, 228.1866) ccw
  arc A26 (587.4541, 221.4671) -> (591.1381, 225.0026) centre (586.4317, 226.2196) ccw
  arc A27 (605.3824, 280.0857) -> (605.7019, 285.9589) centre (590.9592, 283.8155) ccw
  arc A28 (659.4472, 166.7341) -> (664.3899, 169.8264) centre (655.5553, 178.451) ccw
  arc A29 (646.3219, 165.3826) -> (650.9437, 163.9096) centre (649.6446, 167.8208) ccw
  arc A30 (625.7924, 267.3045) -> (622.2982, 265.6147) centre (624.762, 264.9776) ccw
  arc A31 (610.1441, 218.6145) -> (611.1678, 213.2913) centre (616.2651, 217.0316) ccw
  arc A32 (717.0837, 223.8031) -> (716.4363, 227.1645) centre (715.5924, 225.2589) ccw
  arc A33 (576.7137, 198.699) -> (572.0877, 195.5915) centre (578.2952, 191.3476) ccw
  arc A34 (569.9828, 192.5127) -> (568.0661, 187.0445) centre (579.1977, 186.2128) ccw
  arc A35 (596.0683, 200.0622) -> (591.3606, 201.85) centre (592.3346, 197.3225) ccw
  arc A36 (561.488, 99.0072) -> (563.8992, 94.5808) centre (566.1211, 98.661) ccw
  arc A37 (607.161, 71.0227) -> (610.6461, 72.4649) centre (608.3207, 73.1523) ccw
  arc A38 (632.4953, 146.3829) -> (631.5709, 151.6786) centre (626.6918, 148.0984) ccw
  arc A39 (369.3723, 21.5665) -> (373.9863, 24.0953) centre (369.3723, 27.04) ccw
  arc A40 (359.1998, 24.5058) -> (362.8002, 21.5665) centre (362.8002, 25.2412) ccw
  arc A41 (440.2889, 127.9828) -> (439.9093, 132.7535) centre (436.9447, 130.1171) ccw
  arc A42 (424.6176, 149.9496) -> (420.0634, 150.6284) centre (421.9342, 147.5634) ccw
  arc A43 (345.6021, 105.1777) -> (343.6418, 100.6753) centre (347.8283, 101.5304) ccw
  arc A44 (480.0308, 105.8825) -> (479.2087, 109.1906) centre (476.4921, 106.7594) ccw
  arc A45 (479.2087, 109.1906) -> (476.1489, 111.3823) centre (472.7599, 103.4192) ccw
  arc A46 (461.0356, 117.8144) -> (456.6612, 116.4603) centre (459.648, 114.5541) ccw
  arc A47 (397.7124, 24.0953) -> (399.0984, 21.5665) centre (399.0984, 23.2108) ccw
  arc A48 (456.1374, 21.5665) -> (459.859, 24.4784) centre (456.1374, 25.4006) ccw
  arc A49 (612.5479, 21.5665) -> (614.6761, 24.437) centre (612.5479, 23.7907) ccw
  arc A50 (608.3719, 45.1945) -> (604.8654, 49.4997) centre (601.3616, 43.0654) ccw
  arc A51 (549.4168, 79.6941) -> (543.9415, 82.0939) centre (532.6897, 48.9768) ccw
  arc A52 (501.402, 96.5471) -> (497.8399, 94.6002) centre (500.5153, 93.9373) ccw
  arc A53 (480.4639, 24.4784) -> (482.7423, 21.5665) centre (482.7423, 23.9138) ccw
  arc A54 (655.297, 144.2811) -> (651.5996, 140.4585) centre (657.1075, 138.8305) ccw
  arc A55 (742.7191, 106.5435) -> (740.3296, 111.3574) centre (736.6754, 106.5435) ccw
  arc A56 (669.9503, 147.0121) -> (664.3656, 147.2934) centre (666.7965, 139.9751) ccw
  arc A57 (729.4931, 119.5832) -> (724.3659, 122.624) centre (713.6476, 98.7088) ccw
  arc A58 (627.1682, 57.8049) -> (627.1896, 52.0574) centre (636.7694, 54.9669) ccw
  arc A59 (635.5782, 24.437) -> (639.45, 21.5665) centre (639.45, 25.6129) ccw
  arc A60 (739.7191, 21.5665) -> (742.7191, 24.5665) centre (739.7191, 24.5665) ccw
  arc A61 (742.2963, 220.7093) -> (741.5615, 220.2462) centre (742.8959, 218.9435) ccw
  arc A62 (742.7191, 220.4063) -> (742.2963, 220.7093) centre (742.3992, 220.4063) ccw
  arc A63 (741.845, 195.9124) -> (742.7191, 201.7822) centre (722.5746, 201.7822) ccw
  arc A64 (687.0116, 164.3682) -> (687.6536, 160.9946) centre (688.51, 162.9055) ccw
  arc A65 (723.2394, 145.0457) -> (726.8512, 146.6886) centre (724.3211, 147.4593) ccw
  arc A66 (734.1279, 241.2034) -> (739.7116, 240.9533) centre (737.2401, 248.2315) ccw
  arc A67 (739.8784, 241.0099) -> (742.7191, 244.9746) centre (738.5321, 244.9746) ccw
  arc A68 (620.2902, 343.6464) -> (617.837, 341.5008) centre (619.7577, 341.78) ccw
  arc A69 (624.9886, 292.3113) -> (628.1633, 288.1278) centre (630.3618, 293.0925) ccw
  arc A70 (742.7191, 305.7112) -> (739.8343, 309.5344) centre (738.7433, 305.7112) ccw
  arc A71 (604.0386, 382.628) -> (602.9151, 380.6952) centre (604.1846, 381.2502) ccw
  arc A72 (602.9151, 380.6952) -> (604.7133, 377.3815) centre (623.2477, 389.5841) ccw
  arc A73 (609.9478, 369.4309) -> (614.4823, 366.102) centre (616.7009, 373.877) ccw
  arc A74 (742.7191, 394.3219) -> (739.7358, 397.0058) centre (740.0202, 394.3219) ccw
  arc A75 (739.8343, 330.3328) -> (742.7191, 332.5096) centre (740.4554, 332.5096) ccw
  arc A76 (740.1772, 417.1645) -> (742.7191, 419.99) centre (739.8778, 419.99) ccw
  arc A77 (742.7191, 419.99) -> (740.653, 424.0511) centre (737.6948, 419.99) ccw
  arc A78 (583.4317, 418.753) -> (583.4238, 413.8766) centre (586.8289, 416.3094) ccw
  arc A79 (590.5272, 403.9342) -> (595.2545, 401.8092) centre (594.7125, 406.9243) ccw
  arc A80 (642.4132, 495.6115) -> (638.2365, 494.9425) centre (640.6574, 493.2011) ccw
  arc A81 (676.0626, 508.6078) -> (670.2609, 507.1974) centre (680.2694, 478.6651) ccw
  arc A82 (666.4875, 505.8738) -> (666.0815, 503.1144) centre (667.0089, 504.3875) ccw
  arc A83 (742.7191, 514.9727) -> (739.7483, 517.5553) centre (740.1111, 514.9727) ccw
  arc A84 (740.2942, 449.056) -> (742.7191, 450.2896) centre (741.1929, 450.2896) ccw
  arc A85 (742.7191, 641.1318) -> (739.7401, 644.486) centre (739.3413, 641.1318) ccw
  arc A86 (735.8698, 644.9462) -> (731.7682, 642.5184) centre (735.4066, 641.0502) ccw
  arc A87 (687.5923, 533.0484) -> (689.4404, 530.6837) centre (689.1993, 532.3998) ccw
  arc A88 (739.7483, 537.7517) -> (742.7191, 541.1691) centre (739.2682, 541.1691) ccw
  arc A89 (656.1628, 748.7102) -> (656.0297, 748.5263) centre (656.1612, 748.5712) ccw
  arc A90 (741.3477, 664.4358) -> (742.7191, 665.6538) centre (741.4925, 665.6538) ccw
  arc A91 (726.1851, 667.0226) -> (731.9492, 665.5533) centre (734.633, 688.1242) ccw
  arc A92 (676.1888, 689.4893) -> (679.9433, 685.5352) centre (682.3715, 691.6005) ccw
  arc A93 (561.1313, 632.8956) -> (563.0411, 628.7146) centre (564.578, 631.9433) ccw
  arc A94 (636.6347, 743.4339) -> (632.6322, 745.5202) centre (633.5387, 742.3767) ccw
  arc A95 (656.2586, 678.3539) -> (657.0613, 683.6136) centre (651.6146, 681.7538) ccw
  arc A96 (602.5106, 609.9271) -> (606.9916, 611.0584) centre (604.0679, 613.1988) ccw
  arc A97 (600.8806, 586.0695) -> (597.3359, 590.2401) centre (594.4646, 584.2081) ccw
  arc A98 (506.8748, 436.5188) -> (509.0566, 433.287) centre (509.3474, 435.8357) ccw
  arc A99 (557.6326, 609.1389) -> (554.1249, 607.5366) centre (556.5509, 606.8663) ccw
  arc A100 (561.7019, 427.2783) -> (566.4344, 429.3734) centre (562.282, 432.3604) ccw
  arc A101 (621.6245, 506.0985) -> (622.5404, 511.415) centre (616.621, 509.6976) ccw
  arc A102 (581.7776, 372.7675) -> (582.2687, 377.9931) centre (577.3061, 375.8236) ccw
  arc A103 (579.9825, 383.2224) -> (577.0369, 388.4122) centre (553.6748, 371.7213) ccw
  arc A104 (455.7575, 251.5037) -> (457.9483, 248.3641) centre (458.1538, 250.8416) ccw
  arc A105 (565.5679, 404.4652) -> (560.8432, 407.2464) centre (560.0782, 400.5431) ccw
  arc A106 (491.6828, 245.566) -> (496.3653, 247.7948) centre (492.109, 250.7038) ccw
  arc A107 (503.6649, 413.7725) -> (499.8854, 411.221) centre (503.2671, 410.2867) ccw
  arc A108 (501.2387, 219.0357) -> (499.0794, 223.5501) centre (496.7468, 219.6607) ccw
  arc A109 (499.0712, 223.5549) -> (493.5087, 225.3459) centre (492.4435, 212.5037) ccw
  arc A110 (452.5278, 228.745) -> (448.7391, 226.1013) centre (452.2285, 225.1372) ccw
  arc A111 (477.897, 132.3743) -> (482.4785, 133.5835) centre (479.4093, 135.9279) ccw
  arc A112 (433.8983, 191.3463) -> (432.4739, 186.2557) centre (439.6967, 186.9792) ccw
  arc A113 (433.8731, 172.2873) -> (436.1657, 167.0604) centre (443.0806, 173.2096) ccw
  arc A114 (489.0583, 142.1974) -> (491.2928, 147.5528) centre (479.9883, 149.1257) ccw
  arc A115 (458.3883, 142.0703) -> (463.1422, 138.6537) centre (468.3763, 150.9523) ccw
  arc A116 (412.8018, 169.6274) -> (413.8319, 171.699) centre (411.6695, 171.4824) ccw
  arc A117 (413.8319, 171.699) -> (412.5284, 172.3642) centre (412.9662, 171.6123) ccw
  arc A118 (307.1311, 155.8766) -> (305.0939, 152.7557) centre (307.3494, 153.5087) ccw
  arc A119 (329.6477, 122.0713) -> (334.6897, 121.9482) centre (332.2642, 125.9219) ccw
  arc A120 (310.1898, 137.4931) -> (313.6212, 132.9614) centre (318.6111, 140.3048) ccw
  arc A121 (284.6381, 150.8703) -> (280.7006, 153.4406) centre (281.048, 149.6717) ccw
  arc A122 (288.1088, 131.2188) -> (289.7373, 135.5977) centre (286.2061, 134.4187) ccw
  arc A123 (190.5482, 76.2128) -> (193.0344, 74.6849) centre (192.1922, 76.1013) ccw
  arc A124 (304.8483, 114.7423) -> (299.7884, 114.8951) centre (302.1982, 110.8423) ccw
  arc A125 (204.9317, 24.1527) -> (209.8758, 21.5665) centre (209.8758, 27.5852) ccw
  arc A126 (323.4552, 99.5674) -> (320.3734, 104.1928) centre (316.2273, 98.091) ccw
  arc A127 (195.3461, 52.7908) -> (193.5231, 48.1935) centre (197.4159, 49.31) ccw
  arc A128 (336.3872, 21.5665) -> (338.7869, 24.5058) centre (336.3872, 24.0157) ccw
  line L113 (197.4988, 1.5665) -> (762.7191, 1.5665)
  line L114 (762.7191, 1.5665) -> (762.7191, 667.0349)
  arc A129 (762.7191, 667.0349) -> (662.5091, 768.6254) centre (661.1191, 667.0349) ccw
  line L115 (662.5091, 768.6254) -> (656.633, 768.7058)
  arc A130 (656.633, 768.7058) -> (557.312, 694.1724) centre (655.2429, 667.1153) ccw
  line L116 (557.312, 694.1724) -> (426.5564, 220.9132)
  arc A131 (380.9487, 182.765) -> (426.5564, 220.9132) centre (376.1491, 234.8401) ccw
  line L117 (380.9487, 182.765) -> (262.6363, 171.8604)
  arc A132 (262.6363, 171.8604) -> (197.4988, 1.5665) centre (271.961, 70.6892) ccw
  constraint tangent L74 A1
  constraint tangent A0 L74
  constraint tangent A0 L78
  constraint tangent A2 L82
  constraint tangent L101 A3
sketch "Voronoi Sites Sketch" plane through (0, 0, 0) normal (0, 1, 0) x (1, 0, 0)
  point P0 (279.483, 70.5261)
  point P1 (669.8456, 225.7219)
  point P2 (686.7943, 603.4963)
  point P3 (718.5151, 590.6956)
  point P4 (509.3538, 45.9614)
  point P5 (240.8869, 135.4341)
  point P6 (736.7085, 461.2012)
  point P7 (715.859, 432.5785)
  point P8 (709.3762, 106.7101)
  point P9 (694.289, 280.9197)
  point P10 (591.8113, 673.0333)
  point P11 (394.8892, 94.0984)
  point P12 (538.1887, 560.3808)
  point P13 (748.5759, 158.3507)
  point P14 (721.7364, 377.1081)
  point P15 (347.8575, 171.1496)
  point P16 (544.9584, 150.7553)
  point P17 (565.58, 149.2145)
  point P18 (734.0822, 721.6139)
  point P19 (734.4491, 162.6538)
  point P20 (445.5347, 61.7756)
  point P21 (498.505, 186.2395)
  point P22 (514.7248, 183.9827)
  point P23 (542.0093, 258.78)
  point P24 (506.5328, 283.0263)